Autodesk Inventor part; units mm, degrees
(part 2 of 2)
  spline S79 degree 2 poles (165.7626, 207.697) (166.2814, 207.697) (166.906, 208.3921) (166.906, 208.9663) knots 0 0 0 1 2 2 2
  line L364 (166.906, 208.9663) -> (166.906, 210.7646)
  spline S80 degree 2 poles (166.906, 210.7646) (166.906, 211.2784) (166.2663, 211.903) (165.7374, 211.903) knots 0 0 0 1 2 2 2
  spline S81 degree 2 poles (165.7374, 211.903) (165.2186, 211.898) (164.594, 211.2381) (164.594, 210.6488) knots 0 0 0 1 2 2 2
  line L365 (164.594, 210.6488) -> (164.594, 210.4624)
  line L366 (164.594, 210.4624) -> (165.677, 210.4624)
  line L367 (165.677, 210.4624) -> (165.677, 209.5003)
  line L368 (193.4512, 212.85) -> (193.4512, 206.75)
  line L369 (193.4512, 206.75) -> (192.4488, 206.75)
  line L370 (192.4488, 206.75) -> (192.4488, 212.85)
  line L371 (192.4488, 212.85) -> (193.4512, 212.85)
  line L372 (190.0512, 212.85) -> (190.0512, 206.75)
  line L373 (190.0512, 206.75) -> (189.0488, 206.75)
  line L374 (189.0488, 206.75) -> (189.0488, 212.85)
  line L375 (189.0488, 212.85) -> (190.0512, 212.85)
  line L376 (192.9223, 210.3163) -> (192.9223, 209.3542)
  line L377 (192.9223, 209.3542) -> (189.4517, 209.3542)
  line L378 (189.4517, 209.3542) -> (189.4517, 210.3163)
  line L379 (189.4517, 210.3163) -> (192.9223, 210.3163)
  spline S82 degree 2 poles (209.8, 194.8194) (210.4532, 194.8194) (211.4301, 194.3396) (211.9734, 193.4668) (211.9734, 192.8772) knots 0 0 0 1 2 3 3 3
  line L380 (211.9734, 192.8772) -> (211.9734, 192.7616)
  spline S83 degree 2 poles (211.9734, 192.7616) (211.9734, 192.2355) (211.4185, 191.3107) (210.9618, 191.0737) knots 0 0 0 1 2 2 2
  spline S84 degree 2 poles (210.9618, 191.0737) (211.3491, 190.8714) (211.8289, 190.1142) (211.8289, 189.6922) knots 0 0 0 1 2 2 2
  line L381 (211.8289, 189.6922) -> (211.8289, 189.5188)
  spline S85 degree 2 poles (211.8289, 189.5188) (211.8289, 188.6806) (210.7133, 187.6749) (209.8, 187.6749) knots 0 0 0 1 2 2 2
  spline S86 degree 2 poles (209.8, 187.6749) (208.8867, 187.6749) (207.7711, 188.6806) (207.7711, 189.5188) knots 0 0 0 1 2 2 2
  line L382 (207.7711, 189.5188) -> (207.7711, 189.6922)
  spline S87 degree 2 poles (207.7711, 189.6922) (207.7711, 190.1199) (208.2566, 190.8772) (208.6555, 191.0737) knots 0 0 0 1 2 2 2
  spline S88 degree 2 poles (208.6555, 191.0737) (208.1931, 191.3107) (207.6266, 192.2355) (207.6266, 192.7616) knots 0 0 0 1 2 2 2
  line L383 (207.6266, 192.7616) -> (207.6266, 192.8772)
  spline S89 degree 2 poles (207.6266, 192.8772) (207.6266, 193.4668) (208.1757, 194.3396) (209.1468, 194.8194) (209.8, 194.8194) knots 0 0 0 1 2 3 3 3
  spline S90 degree 2 poles (209.8, 193.7153) (209.3376, 193.7153) (208.7769, 193.1777) (208.7769, 192.7442) knots 0 0 0 1 2 2 2
  line L384 (208.7769, 192.7442) -> (208.7769, 192.6749)
  spline S91 degree 2 poles (208.7769, 192.6749) (208.7769, 192.2529) (209.3376, 191.7384) (209.8, 191.7384) knots 0 0 0 1 2 2 2
  spline S92 degree 2 poles (209.8, 191.7384) (210.2566, 191.7384) (210.8289, 192.2529) (210.8231, 192.6806) knots 0 0 0 1 2 2 2
  line L385 (210.8231, 192.6806) -> (210.8231, 192.75)
  spline S93 degree 2 poles (210.8231, 192.75) (210.8231, 193.1835) (210.2624, 193.7153) (209.8, 193.7153) knots 0 0 0 1 2 2 2
  spline S94 degree 2 poles (209.8, 190.6344) (209.4069, 190.6286) (208.9272, 190.1257) (208.9272, 189.7153) knots 0 0 0 1 2 2 2
  line L386 (208.9272, 189.7153) -> (208.9272, 189.646)
  spline S95 degree 2 poles (208.9272, 189.646) (208.9272, 189.2587) (209.4069, 188.7847) (209.8, 188.7847) knots 0 0 0 1 2 2 2
  spline S96 degree 2 poles (209.8, 188.7847) (210.1931, 188.7847) (210.6786, 189.2587) (210.6786, 189.6517) knots 0 0 0 1 2 2 2
  line L387 (210.6786, 189.6517) -> (210.6786, 189.7211)
  spline S97 degree 2 poles (210.6786, 189.7211) (210.6786, 190.1373) (210.1931, 190.6344) (209.8, 190.6344) knots 0 0 0 1 2 2 2
  line L388 (207.8954, 162.25) -> (207.8954, 163.1228)
  line L389 (207.8954, 163.1228) -> (209.589, 169.25)
  line L390 (209.589, 169.25) -> (210.826, 169.25)
  line L391 (210.826, 169.25) -> (209.1555, 163.354)
  line L392 (209.1555, 163.354) -> (210.6526, 163.354)
  line L393 (210.6526, 163.354) -> (210.6526, 164.3829)
  line L394 (210.6526, 164.3829) -> (211.8029, 164.3829)
  line L395 (211.8029, 164.3829) -> (211.8029, 162.25)
  line L396 (211.8029, 162.25) -> (207.8954, 162.25)
  spline S98 degree 2 poles (209.8087, 118.2818) (210.6237, 118.2818) (211.7104, 117.276) (211.8087, 116.3627) knots 0 0 0 1 2 2 2
  line L397 (211.8087, 116.3627) -> (211.8087, 116.3512)
  line L398 (211.8087, 116.3512) -> (210.6584, 116.3512)
  line L399 (210.6584, 116.3512) -> (210.6584, 116.3569)
  spline S99 degree 2 poles (210.6584, 116.3569) (210.6179, 116.7442) (210.1613, 117.172) (209.7971, 117.172) knots 0 0 0 1 2 2 2
  spline S100 degree 2 poles (209.7971, 117.172) (209.3867, 117.172) (208.9416, 116.6286) (208.9416, 116.1373) knots 0 0 0 1 2 2 2
  line L400 (208.9416, 116.1373) -> (208.9416, 115.5477)
  spline S101 degree 2 poles (208.9416, 115.5477) (208.9416, 115.0564) (209.3636, 114.5188) (209.7624, 114.5188) knots 0 0 0 1 2 2 2
  spline S102 degree 2 poles (209.7624, 114.5188) (210.0283, 114.5188) (210.4618, 114.8078) (210.5948, 115.0679) knots 0 0 0 1 2 2 2
  line L401 (210.5948, 115.0679) -> (211.6584, 115.0679)
  line L402 (211.6584, 115.0679) -> (211.6584, 111.2124)
  line L403 (211.6584, 111.2124) -> (207.9936, 111.2124)
  line L404 (207.9936, 111.2124) -> (207.9936, 112.3165)
  line L405 (207.9936, 112.3165) -> (210.5081, 112.3165)
  line L406 (210.5081, 112.3165) -> (210.5081, 113.7211)
  spline S103 degree 2 poles (210.5081, 113.7211) (210.3347, 113.5708) (209.8491, 113.409) (209.6121, 113.409) knots 0 0 0 1 2 2 2
  spline S104 degree 2 poles (209.6121, 113.409) (208.7451, 113.409) (207.7913, 114.5303) (207.7913, 115.5477) knots 0 0 0 1 2 2 2
  line L407 (207.7913, 115.5477) -> (207.7913, 116.1373)
  spline S105 degree 2 poles (207.7913, 116.1373) (207.7913, 117.1604) (208.8491, 118.2818) (209.8087, 118.2818) knots 0 0 0 1 2 2 2
  line L408 (212.3467, 92.0147) -> (212.3467, 90.8322)
  line L409 (212.3467, 90.8322) -> (209.7703, 85.25)
  line L410 (209.7703, 85.25) -> (208.3434, 85.25)
  line L411 (208.3434, 85.25) -> (210.8471, 90.7661)
  line L412 (210.8471, 90.7661) -> (207.0948, 90.7661)
  line L413 (207.0948, 90.7661) -> (207.0948, 92.0147)
  line L414 (207.0948, 92.0147) -> (212.3467, 92.0147)
  line L415 (209.004, 93.25) -> (209.004, 88.5398)
  line L416 (209.004, 88.5398) -> (207.7026, 88.5398)
  line L417 (207.7026, 88.5398) -> (207.7026, 93.25)
  line L418 (207.7026, 93.25) -> (209.004, 93.25)
  spline S106 degree 2 poles (209.852, 67.3194) (210.459, 67.3194) (211.4012, 66.8743) (211.9618, 66.0303) (212.0197, 65.435) knots 0 0 0 1 2 3 3 3
  line L419 (212.0197, 65.435) -> (210.8347, 65.435)
  spline S107 degree 2 poles (210.8347, 65.435) (210.7769, 65.8223) (210.2971, 66.2095) (209.9214, 66.2095) knots 0 0 0 1 2 2 2
  spline S108 degree 2 poles (209.9214, 66.2095) (209.4879, 66.2095) (209.0197, 65.7355) (209.0197, 65.3136) knots 0 0 0 1 2 2 2
  line L420 (209.0197, 65.3136) -> (209.0197, 65.1286)
  spline S109 degree 2 poles (209.0197, 65.1286) (209.0197, 64.6662) (209.4358, 64.1575) (209.8231, 64.1575) knots 0 0 0 1 2 2 2
  line L421 (209.8231, 64.1575) -> (210.3723, 64.1575)
  line L422 (210.3723, 64.1575) -> (210.3723, 63.0535)
  line L423 (210.3723, 63.0535) -> (209.8231, 63.0535)
  spline S110 degree 2 poles (209.8231, 63.0535) (209.4936, 63.0535) (209.1353, 62.6199) (209.1353, 62.2269) knots 0 0 0 1 2 2 2
  line L424 (209.1353, 62.2269) -> (209.1353, 62.0592)
  spline S111 degree 2 poles (209.1353, 62.0592) (209.1353, 61.6893) (209.5225, 61.2905) (209.8809, 61.2905) knots 0 0 0 1 2 2 2
  spline S112 degree 2 poles (209.8809, 61.2905) (210.1988, 61.2905) (210.6439, 61.7009) (210.7249, 62.1113) knots 0 0 0 1 2 2 2
  line L425 (210.7249, 62.1113) -> (211.904, 62.1113)
  spline S113 degree 2 poles (211.904, 62.1113) (211.7884, 61.1864) (210.6786, 60.1749) (209.852, 60.1749) knots 0 0 0 1 2 2 2
  spline S114 degree 2 poles (209.852, 60.1749) (208.9329, 60.1749) (207.9329, 61.1228) (207.9329, 61.9957) knots 0 0 0 1 2 2 2
  line L426 (207.9329, 61.9957) -> (207.9329, 62.1633)
  spline S115 degree 2 poles (207.9329, 62.1633) (207.9329, 62.6662) (208.4647, 63.4118) (208.9503, 63.5968) knots 0 0 0 1 2 2 2
  spline S116 degree 2 poles (208.9503, 63.5968) (208.4127, 63.7124) (207.8173, 64.5679) (207.8173, 65.2269) knots 0 0 0 1 2 2 2
  line L427 (207.8173, 65.2269) -> (207.8173, 65.3887)
  spline S117 degree 2 poles (207.8173, 65.3887) (207.8173, 66.3136) (208.8809, 67.3194) (209.852, 67.3194) knots 0 0 0 1 2 2 2
  line L428 (211.7827, 41.7876) -> (211.7827, 40.7645)
  line L429 (211.7827, 40.7645) -> (209.3607, 37.5621)
  spline S118 degree 2 poles (209.3607, 37.5621) (209.1699, 37.3136) (208.9618, 36.7876) (208.9618, 36.5621) knots 0 0 0 1 2 2 2
  line L430 (208.9618, 36.5621) -> (208.9618, 36.5564)
  spline S119 degree 2 poles (208.9618, 36.5564) (208.9618, 36.2038) (209.3954, 35.8165) (209.7884, 35.8165) knots 0 0 0 1 2 2 2
  spline S120 degree 2 poles (209.7884, 35.8165) (210.1584, 35.8165) (210.6324, 36.2847) (210.6844, 36.7124) knots 0 0 0 1 2 2 2
  line L431 (210.6844, 36.7124) -> (210.6844, 36.7182)
  line L432 (210.6844, 36.7182) -> (211.8694, 36.7182)
  line L433 (211.8694, 36.7182) -> (211.8694, 36.7124)
  spline S121 degree 2 poles (211.8694, 36.7124) (211.7653, 35.7587) (210.6671, 34.7124) (209.7942, 34.7124) knots 0 0 0 1 2 2 2
  spline S122 degree 2 poles (209.7942, 34.7124) (208.8289, 34.7124) (207.7769, 35.6662) (207.7769, 36.539) knots 0 0 0 1 2 2 2
  line L434 (207.7769, 36.539) -> (207.7769, 36.5448)
  spline S123 degree 2 poles (207.7769, 36.5448) (207.7769, 36.9668) (208.0948, 37.8454) (208.3838, 38.2211) knots 0 0 0 1 2 2 2
  line L435 (208.3838, 38.2211) -> (210.2566, 40.6835)
  line L436 (210.2566, 40.6835) -> (207.7364, 40.6835)
  line L437 (207.7364, 40.6835) -> (207.7364, 41.7876)
  line L438 (207.7364, 41.7876) -> (211.7827, 41.7876)
  line L439 (208.9763, 9.25) -> (208.9763, 16.25)
  line L440 (208.9763, 16.25) -> (210.1266, 16.25)
  line L441 (210.1266, 16.25) -> (210.1266, 10.5564)
  line L442 (210.1266, 10.5564) -> (211.0514, 11.0246)
  line L443 (211.0514, 11.0246) -> (211.0514, 9.8165)
  line L444 (211.0514, 9.8165) -> (210.0341, 9.25)
  line L445 (210.0341, 9.25) -> (208.9763, 9.25)
  line L446 (192.4488, -8.8562) -> (192.4488, -2.7562)
  line L447 (192.4488, -2.7562) -> (193.4512, -2.7562)
  line L448 (193.4512, -2.7562) -> (193.4512, -8.8562)
  line L449 (193.4512, -8.8562) -> (192.4488, -8.8562)
  line L450 (189.0488, -8.8562) -> (189.0488, -2.7562)
  line L451 (189.0488, -2.7562) -> (190.0512, -2.7562)
  line L452 (190.0512, -2.7562) -> (190.0512, -8.8562)
  line L453 (190.0512, -8.8562) -> (189.0488, -8.8562)
  line L454 (189.5777, -6.3225) -> (189.5777, -5.3604)
  line L455 (189.5777, -5.3604) -> (193.0483, -5.3604)
  line L456 (193.0483, -5.3604) -> (193.0483, -6.3225)
  line L457 (193.0483, -6.3225) -> (189.5777, -6.3225)
  line L458 (165.823, -5.5003) -> (167.9386, -5.5003)
  line L459 (167.9386, -5.5003) -> (167.9386, -6.6286)
  spline S124 degree 2 poles (167.9386, -6.6286) (167.9386, -7.3187) (167.3946, -8.3463) (166.4225, -8.9104) (165.7626, -8.9104) knots 0 0 0 1 2 3 3 3
  spline S125 degree 2 poles (165.7626, -8.9104) (165.1027, -8.9104) (164.1104, -8.3815) (163.5614, -7.4094) (163.5614, -6.7646) knots 0 0 0 1 2 3 3 3
  line L460 (163.5614, -6.7646) -> (163.5614, -4.9663)
  spline S126 degree 2 poles (163.5614, -4.9663) (163.5614, -4.2763) (164.1054, -3.2537) (165.0826, -2.6845) (165.7374, -2.6845) knots 0 0 0 1 2 3 3 3
  spline S127 degree 2 poles (165.7374, -2.6845) (166.2764, -2.6845) (167.173, -3.1379) (167.7825, -3.9539) (167.8883, -4.4979) knots 0 0 0 1 2 3 3 3
  line L461 (167.8883, -4.4979) -> (166.8053, -4.4979)
  spline S128 degree 2 poles (166.8053, -4.4979) (166.7045, -4.1151) (166.09, -3.697) (165.7374, -3.697) knots 0 0 0 1 2 2 2
  spline S129 degree 2 poles (165.7374, -3.697) (165.2186, -3.697) (164.594, -4.3921) (164.594, -4.9663) knots 0 0 0 1 2 2 2
  line L462 (164.594, -4.9663) -> (164.594, -6.7646)
  spline S130 degree 2 poles (164.594, -6.7646) (164.594, -7.2784) (165.2337, -7.903) (165.7626, -7.903) knots 0 0 0 1 2 2 2
  spline S131 degree 2 poles (165.7626, -7.903) (166.2814, -7.898) (166.906, -7.2381) (166.906, -6.6488) knots 0 0 0 1 2 2 2
  line L463 (166.906, -6.6488) -> (166.906, -6.4624)
  line L464 (166.906, -6.4624) -> (165.823, -6.4624)
  line L465 (165.823, -6.4624) -> (165.823, -5.5003)
  line L466 (138.5626, -8.85) -> (138.5626, -2.75)
  line L467 (138.5626, -2.75) -> (139.5649, -2.75)
  line L468 (139.5649, -2.75) -> (139.5649, -8.85)
  line L469 (139.5649, -8.85) -> (138.5626, -8.85)
  line L470 (138.9806, -3.7121) -> (138.9806, -2.75)
  line L471 (138.9806, -2.75) -> (142.4815, -2.75)
  line L472 (142.4815, -2.75) -> (142.4815, -3.7121)
  line L473 (142.4815, -3.7121) -> (138.9806, -3.7121)
  line L474 (138.9806, -6.3516) -> (138.9806, -5.3945)
  line L475 (138.9806, -5.3945) -> (142.0231, -5.3945)
  line L476 (142.0231, -5.3945) -> (142.0231, -6.3516)
  line L477 (142.0231, -6.3516) -> (138.9806, -6.3516)
  line L478 (112.8963, -8.85) -> (112.8963, -2.75)
  line L479 (112.8963, -2.75) -> (113.8987, -2.75)
  line L480 (113.8987, -2.75) -> (113.8987, -8.85)
  line L481 (113.8987, -8.85) -> (112.8963, -8.85)
  line L482 (113.3094, -3.7121) -> (113.3094, -2.75)
  line L483 (113.3094, -2.75) -> (116.8958, -2.75)
  line L484 (116.8958, -2.75) -> (116.8958, -3.7121)
  line L485 (116.8958, -3.7121) -> (113.3094, -3.7121)
  line L486 (113.3094, -8.85) -> (113.3094, -7.8879)
  line L487 (113.3094, -7.8879) -> (116.8958, -7.8879)
  line L488 (116.8958, -7.8879) -> (116.8958, -8.85)
  line L489 (116.8958, -8.85) -> (113.3094, -8.85)
  line L490 (113.3094, -6.3012) -> (113.3094, -5.3391)
  line L491 (113.3094, -5.3391) -> (116.4374, -5.3441)
  line L492 (116.4374, -5.3441) -> (116.4374, -6.3012)
  line L493 (116.4374, -6.3012) -> (113.3094, -6.3012)
  line L494 (87.7237, -8.85) -> (87.7237, -7.8879)
  line L495 (87.7237, -7.8879) -> (89.1442, -7.8879)
  spline S132 degree 2 poles (89.1442, -7.8879) (89.7638, -7.8879) (90.4488, -7.2633) (90.4488, -6.6991) knots 0 0 0 1 2 2 2
  line L496 (90.4488, -6.6991) -> (90.4488, -4.9009)
  spline S133 degree 2 poles (90.4488, -4.9009) (90.4488, -4.3317) (89.7638, -3.7121) (89.1442, -3.7121) knots 0 0 0 1 2 2 2
  line L497 (89.1442, -3.7121) -> (87.7237, -3.7121)
  line L498 (87.7237, -3.7121) -> (87.7237, -2.75)
  line L499 (87.7237, -2.75) -> (89.119, -2.75)
  spline S134 degree 2 poles (89.119, -2.75) (90.2474, -2.75) (91.4815, -3.8934) (91.4815, -4.9361) knots 0 0 0 1 2 2 2
  line L500 (91.4815, -4.9361) -> (91.4815, -6.6639)
  spline S135 degree 2 poles (91.4815, -6.6639) (91.4815, -7.3338) (90.9374, -8.3161) (89.8847, -8.85) (89.114, -8.85) knots 0 0 0 1 2 3 3 3
  line L501 (89.114, -8.85) -> (87.7237, -8.85)
  line L502 (87.1445, -8.85) -> (87.1445, -2.75)
  line L503 (87.1445, -2.75) -> (88.1469, -2.75)
  line L504 (88.1469, -2.75) -> (88.1469, -8.85)
  line L505 (88.1469, -8.85) -> (87.1445, -8.85)
  spline S136 degree 2 poles (63.8407, -8.9104) (63.1758, -8.9104) (62.2036, -8.3614) (61.6797, -7.3389) (61.6797, -6.6387) knots 0 0 0 1 2 3 3 3
  line L506 (61.6797, -6.6387) -> (61.6797, -4.9663)
  spline S137 degree 2 poles (61.6797, -4.9663) (61.6797, -4.2561) (62.2036, -3.2336) (63.1758, -2.6845) (63.8407, -2.6845) knots 0 0 0 1 2 3 3 3
  spline S138 degree 2 poles (63.8407, -2.6845) (64.3948, -2.6845) (65.2863, -3.158) (65.8757, -4.0395) (65.9865, -4.644) knots 0 0 0 1 2 3 3 3
  line L507 (65.9865, -4.644) -> (64.9539, -4.644)
  spline S139 degree 2 poles (64.9539, -4.644) (64.8783, -4.3417) (64.5509, -3.9136) (64.1026, -3.6768) (63.8407, -3.6768) knots 0 0 0 1 2 3 3 3
  spline S140 degree 2 poles (63.8407, -3.6768) (63.3218, -3.6768) (62.7123, -4.3669) (62.7123, -4.9663) knots 0 0 0 1 2 2 2
  line L508 (62.7123, -4.9663) -> (62.7123, -6.6387)
  spline S141 degree 2 poles (62.7123, -6.6387) (62.7123, -7.228) (63.3218, -7.9181) (63.8407, -7.9181) knots 0 0 0 1 2 2 2
  spline S142 degree 2 poles (63.8407, -7.9181) (64.2336, -7.9181) (64.8481, -7.4194) (64.9539, -6.951) knots 0 0 0 1 2 2 2
  line L509 (64.9539, -6.951) -> (65.9865, -6.951)
  spline S143 degree 2 poles (65.9865, -6.951) (65.8757, -7.5554) (65.2813, -8.437) (64.3948, -8.9104) (63.8407, -8.9104) knots 0 0 0 1 2 3 3 3
  point P0 (0, 0)
  point P1 (0.0104, 102.0099)
  point P2 (1.1, -1.1)
  point P3 (179.6, -1.1)
  point P4 (202.9, -10.5)
  point P5 (-1.1, 1.1)
  point P6 (-1.1, 26.6)
  point P7 (-1.1, 52.1)
  point P8 (-1.1, 77.6)
  point P9 (179.6, 3.161)
  point P10 (1.1, 214.5)
  point P11 (24.4, 205.1)
  point P12 (26.6, 214.5)
  point P13 (52.1, 214.5)
  point P14 (214.5, 1.1)
  point P15 (214.5, 26.6)
  dimension "d0" = 25.5
  dimension "d1" = 25.5
  constraints: 102 coincident, 5 point on line, 2 horizontal, 1 vertical, 72 other
extrude "Extrusion10" cut sketch "Sketch10" against normal blind 0.5 contours S0 | S2 | L198 L199 L200 L201 L202 L208 L207 L206 L203 L205 L204 | L208 L205 L206 L203 | L203 L206 L202 L208 | L202 L206 L207 L208 | L223 L220 L221 L216 L215 L222 L214 L213 L212 L210 L209 | L209 L210 L222 L219 | L222 L210 S4 L211 S5 L212 L214 S6 S7 L215 L217 S8 S9 S10 L218 S11 L219 | L212 L213 L214 L222 | L217 L222 L215 L216 | S12 L224 S13 S14 L225 S15 S16 L226 S17 S18 L227 S19 | L232 L233 L234 L235 L236 L237 L238 L239 L240 | S28 L241 L242 L243 S29 S30 L244 S31 S32 L245 L246 L247 L248 L249 L250 S33 S34 L251 S35 | L252 L253 L254 L255 L256 L259 L258 | L259 L256 L261 L258 | L258 L261 L262 L259 | L261 L256 L257 L258 | L259 L260 L261 L256 | S36 L263 S37 S38 L264 S39 L265 L266 L267 S40 L268 S41 S42 L269 S43 S44 L270 S45 S46 L271 S47 | L272 L273 S48 L274 S49 S50 L275 L276 L277 S51 S52 L278 S53 L279 L280 L281 L282 | L283 L284 L285 L286 L287 L288 L289 | L290 L291 L292 L293 L294 L300 L299 L298 L295 L297 L296 | L300 L297 L298 L295 | L295 L298 L294 L300 | L294 L298 L299 L300 | L315 L312 L313 L308 L307 L314 L306 L305 L304 L302 L301 | L301 L302 L314 L311 | L314 L302 S54 L303 S55 L304 L306 S56 S57 L307 L309 S58 S59 S60 L310 S61 L311 | L304 L305 L306 L314 | L309 L314 L307 L308 | S62 L316 S63 S64 L317 S65 S66 L318 S67 S68 L319 S69 | L331 L328 L329 L324 L323 L330 L321 L320 | L320 L321 L330 L327 | L330 L321 S70 L322 S71 L323 L325 S72 L326 S73 L327 | L323 L324 L325 L330 | L332 L333 L336 L339 L334 L345 L344 L347 L341 L340 L335 | L340 L341 L334 L335 | L333 L334 L339 L336 | L334 L341 L342 L343 | L337 L338 L339 L334 | L347 L344 L345 L334 | L334 L345 L346 L347 | L348 L349 L352 L355 L350 L357 L356 L359 L351 | L349 L350 L355 L352 | L359 L356 L357 L350 | L350 L357 L358 L359 | L353 L354 L355 L350 | L360 L361 S74 S75 L362 S76 S77 L363 S78 S79 L364 S80 S81 L365 L366 L367 | L368 L369 L370 L377 L376 L379 L371 | L379 L376 L377 L370 | L370 L377 L372 L379 | L379 L378 L377 L372 L373 L374 L375 | L372 L377 L378 L379 | S82 L380 S83 S84 L381 S85 S86 L382 S87 S88 L383 S89 | L388 L389 L390 L391 L392 L393 L394 L395 L396 | S98 L397 L398 L399 S99 S100 L400 S101 S102 L401 L402 L403 L404 L405 L406 S103 S104 L407 S105 | L408 L409 L410 L411 L412 L415 L414 | L415 L412 L417 L414 | L414 L417 L418 L415 | L417 L412 L413 L414 | L415 L416 L417 L412 | S106 L419 S107 S108 L420 S109 L421 L422 L423 S110 L424 S111 S112 L425 S113 S114 L426 S115 S116 L427 S117 | L428 L429 S118 L430 S119 S120 L431 L432 L433 S121 S122 L434 S123 L435 L436 L437 L438 | L439 L440 L441 L442 L443 L444 L445 | L446 L457 L456 L455 L447 L448 L449 | L457 L452 L455 L446 | L446 L455 L456 L457 | L457 L454 L455 L452 | L452 L453 L450 L451 L455 L454 L457 | L458 L459 S124 S125 L460 S126 S127 L461 S128 S129 L462 S130 S131 L463 L464 L465 | L466 L467 L470 L473 L468 L475 L474 L477 L469 | L467 L468 L473 L470 | L477 L474 L475 L468 | L468 L475 L476 L477 | L471 L472 L473 L468 | L478 L479 L482 L485 L480 L491 L490 L493 L487 L486 L481 | L486 L487 L480 L481 | L479 L480 L485 L482 | L480 L487 L488 L489 | L483 L484 L485 L480 | L493 L490 L491 L480 | L480 L491 L492 L493 | L505 L502 L503 L498 L497 L504 L495 L494 | L494 L495 L504 L501 | L504 L495 S132 L496 S133 L497 L499 S134 L500 S135 L501 | L497 L498 L499 L504 | S136 L506 S137 S138 L507 S139 S140 L508 S141 S142 L509 S143 bodies 2
equation "\"d9\" = 0.5 * d8"
equation "\"d11\" = 0.5 * d10"
